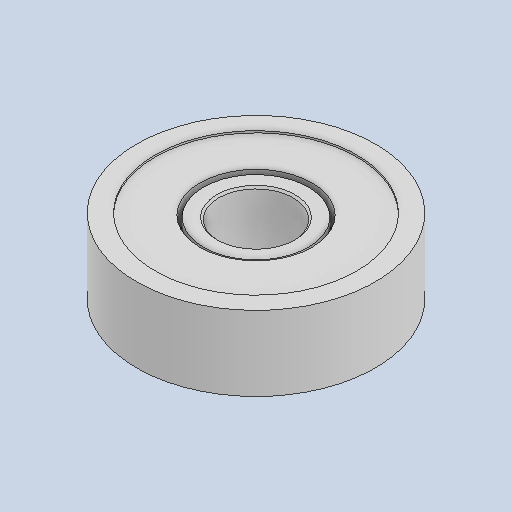
# Autodesk Inventor part: lozysko
Saved by Autodesk Inventor 2025.2 (Build 292293000, 293)
## iProperties
Created: 2025-03-20
Part Number: lozysko
Material: Ogólny
Document SubType Name: Modeling
Designer: tadek
Density: 1 g/cm^3
Appearance: Domyślna
Author: tadek
Autodesk Inventor part; units mm, degrees
ref_plane "YZ Plane" through (0, 0, 0) normal (1, 0, 0) x (0, 1, 0)
ref_plane "XZ Plane" through (0, 0, 0) normal (0, 1, 0) x (-1, 0, 0)
ref_plane "XY Plane" through (0, 0, 0) normal (0, 0, 1) x (1, 0, 0)
sketch "Szkic1" plane through (0, 0, 0) normal (0, 1, 0) x (-1, 0, 0)
  circle A0 centre (0, 0) radius 2.5
  circle A1 centre (0, 0) radius 8
  circle A2 centre (0, 0) radius 3.5
  circle A3 centre (0, 0) radius 3.5
  circle A4 centre (0, 0) radius 6.75
  circle A5 centre (0, 0) radius 5
  circle A6 centre (0, 0) radius 3.75
  dimension "d0" = 5
  dimension "d1" = 16
  dimension "d2" = 7
  dimension "d3" = 7
  dimension "d4" = 13.5
  dimension "d13" = 10
  dimension "d16" = 7.5
  constraints: 7 centre point, 7 coincident
  measures "d0" diameter of A0
  measures "d1" diameter of A1
  measures "d2" diameter of A2
  measures "d3" diameter of A3
  measures "d4" diameter of A4
  measures "d13" diameter of A5
  measures "d16" diameter of A6
extrude "Wyciągnięcie proste7" add sketch "Szkic1" along normal mid plane 4.5 contours A2
extrude "Wyciągnięcie proste8" add sketch "Szkic1" along normal mid plane 4.75 contours A5
extrude "Wyciągnięcie proste9" add sketch "Szkic1" along normal mid plane 1.5 contours A0 | A2 | A6
extrude "Wyciągnięcie proste10" add sketch "Szkic1" along normal mid plane 5 contours A1
extrude "Wyciągnięcie proste11" add sketch "Szkic1" along normal mid plane 4.75 contours A4
sketch "Szkic2" plane through (0, 0.75, 0) normal (0, 1, 0) x (1, 0, 0)
  point P0 (0, 0)
  point P1 (0.0085, 0.051)
hole "Otwór3" at (0, 0.75, 0) direction (0, -1, 0) diameter 5 end through all
chamfer "Faza3" distance 0.125 angle 45 1 edges at (2.5, 2.25, 0)
